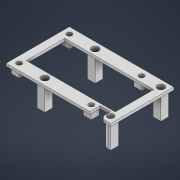
# Autodesk Inventor part: Adapter_Spannungswandler
Saved by Autodesk Inventor 2021 (Build 250183000, 183)
## iProperties
Created: 2021-02-07
Part Number: Adapter_Spannungswandler
Material: Generisch
Document SubType Name: Modeling
Designer: Ctroi
Density: 1 g/cm^3
Appearance: Vorgabe
Author: Ctroi
Autodesk Inventor part; units mm, degrees
ref_plane "YZ Plane" through (0, 0, 0) normal (1, 0, 0) x (0, 1, 0)
ref_plane "XZ Plane" through (0, 0, 0) normal (0, 1, 0) x (-1, 0, 0)
ref_plane "XY Plane" through (0, 0, 0) normal (0, 0, 1) x (1, 0, 0)
sketch "Skizze1" plane through (0, 0, 0) normal (0, 1, 0) x (-1, 0, 0)
  line L0 (28.5, 22.5) -> (-28.5, 22.5)
  line L1 (-28.5, 22.5) -> (-28.5, -22.5)
  line L2 (-28.5, -22.5) -> (28.5, -22.5)
  line L3 (28.5, -22.5) -> (28.5, 22.5)
  line L4 (-39.9, 0) -> (39.9, 0) projected
  line L5 (0, -31.5) -> (0, 31.5) projected
  circle A0 centre (-25.5, 19.5) radius 1.6
  circle A1 centre (25.5, 19.5) radius 1.6
  circle A2 centre (25.5, -19.5) radius 1.6
  circle A3 centre (-25.5, -19.5) radius 1.6
  line L6 (-28.5, 22.5) -> (-22.5, 22.5)
  line L7 (-22.5, 22.5) -> (-22.5, 16.5)
  line L8 (-22.5, 16.5) -> (-28.5, 16.5)
  line L9 (-28.5, 16.5) -> (-28.5, 22.5)
  line L10 (-14.5, 22.5) -> (-22.5, 22.5)
  line L11 (-22.5, 22.5) -> (-22.5, 16.5)
  line L12 (-22.5, 16.5) -> (-14.5, 16.5)
  line L13 (-14.5, 16.5) -> (-14.5, 22.5)
  line L14 (-28.5, -22.5) -> (-22.5, -22.5)
  line L15 (-22.5, -22.5) -> (-22.5, -16.5)
  line L16 (-22.5, -16.5) -> (-28.5, -16.5)
  line L17 (-28.5, -16.5) -> (-28.5, -22.5)
  line L18 (28.5, -22.5) -> (22.5, -22.5)
  line L19 (22.5, -22.5) -> (22.5, -16.5)
  line L20 (22.5, -16.5) -> (28.5, -16.5)
  line L21 (28.5, -16.5) -> (28.5, -22.5)
  line L22 (28.5, 22.5) -> (22.5, 22.5)
  line L23 (22.5, 22.5) -> (22.5, 16.5)
  line L24 (22.5, 16.5) -> (28.5, 16.5)
  line L25 (28.5, 16.5) -> (28.5, 22.5)
  point P0 (0, 0)
  dimension "d0" = 57
  dimension "d1" = 45
  dimension "d2" = 3.2
  dimension "d3" = 3.2
  dimension "d4" = 3.2
  dimension "d5" = 3.2
  dimension "d6" = 39
  dimension "d7" = 19.5
  dimension "d8" = 51
  dimension "d9" = 51
  dimension "d10" = 39
  dimension "d11" = 19.5
  dimension "d13" = 3
  dimension "d14" = 25.5
  dimension "d15" = 6
  dimension "d16" = 6
  dimension "d17" = 0
  dimension "d18" = 8
  dimension "d19" = 6
  dimension "d20" = 6
  dimension "d21" = 6
  dimension "d22" = 6
  dimension "d23" = 6
  dimension "d24" = 6
  constraints: 48 end point, 12 parallel, 6 horizontal, 6 perpendicular, 4 centre point, 2 point on line, 2 other
  measures "d0" distance of L2.end L1.end
  measures "d1" distance of L1.end L0.end
  measures "d2" diameter of A0
  measures "d3" diameter of A1
  measures "d4" diameter of A2
  measures "d5" diameter of A3
  measures "d6" distance of A2.centre A1.centre
  measures "d7" distance from line of L4 A1.centre
  measures "d8" distance of A0.centre A1.centre
  measures "d9" distance of A3.centre A2.centre
  measures "d10" distance of A3.centre A0.centre
  measures "d11" distance from line of L4 A0.centre
  measures "d13" distance from line of L2 A2.centre
  measures "d14" distance from line of L5 A1.centre
  measures "d15" distance of L7.end L8.end
  measures "d16" distance of L6.end L7.end
  measures "d17" distance between parallel lines of L7 L11
  measures "d18" distance between parallel lines of L7 L13
  measures "d19" distance of L16.end L15.end
  measures "d20" distance of L15.end L14.end
  measures "d21" distance of L19.end L20.end
  measures "d22" distance of L18.end L19.end
  measures "d23" distance of L24.end L23.end
  measures "d24" distance of L23.end L22.end
extrude "Extrusion1" add sketch "Skizze1" along normal blind 2 and the other way blind 23 contours L3 L24 L23 L0 | L3 L2 L19 L20 | L7 L8 L1 L0 | L16 L15 L2 L1
extrude "Extrusion2" add sketch "Skizze1" along normal blind 2 contours L23 L24 L3 L4 L5 L0 | L5 L4 L1 L8 L12 L13 L0 | L3 L20 L19 L2 L5 L4 | L5 L2 L15 L16 L1 L4
sketch "Skizze2" plane through (-28.5, -23, 22.5) normal (-1, 0, 0) x (0, 0, 1)
  line L0 (0, 0) -> (0, 25) projected
  line L1 (-45, 0) -> (-45, 25) projected
  line L2 (0, 25) -> (-45, 25)
  line L3 (-45, 25) -> (-45, 23)
  line L4 (-45, 23) -> (0, 23)
  line L5 (0, 23) -> (0, 25)
  point P0 (-22.5, 23)
  constraints: 8 end point, 2 parallel, 1 horizontal, 1 perpendicular, 1 point on line
extrude "Extrusion3" add sketch "Skizze2" along normal blind 20
sketch "Skizze4" plane through (0, 0, 0) normal (0, -1, 0) x (1, 0, 0)
  line L0 (-48.5, 22.5) -> (-48.5, -22.5) projected
  line L1 (-48.5, -22.5) -> (-42.5, -22.5)
  line L2 (-42.5, -22.5) -> (-42.5, -16.5)
  line L3 (-42.5, -16.5) -> (-48.5, -16.5)
  line L4 (-48.5, -16.5) -> (-48.5, -22.5)
  line L5 (-48.5, 22.5) -> (-42.5, 22.5)
  line L6 (-42.5, 22.5) -> (-42.5, 16.5)
  line L7 (-42.5, 16.5) -> (-48.5, 16.5)
  line L8 (-48.5, 16.5) -> (-48.5, 22.5)
  line L9 (22.5, -22.5) -> (-22.5, -22.5) projected
  line L10 (7.5, -22.5) -> (13.5, -22.5)
  line L11 (13.5, -22.5) -> (13.5, -16.5)
  line L12 (13.5, -16.5) -> (7.5, -16.5)
  line L13 (7.5, -16.5) -> (7.5, -22.5)
  line L14 (28.5, 16.5) -> (28.5, -16.5) projected
  line L15 (-22.5, 22.5) -> (14.5, 22.5) projected
  line L16 (13.5, 22.5) -> (7.5, 22.5)
  line L17 (7.5, 22.5) -> (7.5, 16.5)
  line L18 (7.5, 16.5) -> (13.5, 16.5)
  line L19 (13.5, 16.5) -> (13.5, 22.5)
  line L20 (28.5, 16.5) -> (28.5, 22.5) projected
  point P0 (0, 0)
  dimension "d45" = 6
  dimension "d46" = 6
  dimension "d47" = 6
  dimension "d48" = 6
  dimension "d49" = 6
  dimension "d50" = 6
  dimension "d51" = 15
  dimension "d52" = 6
  dimension "d53" = 6
  dimension "d54" = 15
  constraints: 32 end point, 8 parallel, 4 horizontal, 4 perpendicular, 2 point on line
  measures "d45" distance of L3.end L2.end
  measures "d46" distance of L2.end L1.end
  measures "d47" distance of L6.end L7.end
  measures "d48" distance of L5.end L6.end
  measures "d49" distance of L12.end L11.end
  measures "d50" distance of L11.end L10.end
  measures "d51" distance between parallel lines of L14 L11
  measures "d52" distance of L18.end L17.end
  measures "d53" distance of L17.end L16.end
  measures "d54" distance between parallel lines of L20 L19
extrude "Extrusion4" add sketch "Skizze4" along normal blind 5
sketch "Skizze3" plane through (0, 2, 0) normal (0, 1, 0) x (1, 0, 0)
  circle A0 centre (10.5, -19.5) radius 2
  circle A1 centre (10.5, 19.5) radius 2
  line L0 (43.9, 0) -> (-63.9, 0) projected
  line L1 (28.5, -22.5) -> (28.5, 22.5) projected
  circle A2 centre (-45.5, -19.5) radius 2
  circle A3 centre (-45.5, 19.5) radius 2
  line L2 (14.5, -22.5) -> (-48.5, -22.5) projected
  line L3 (28.5, 22.5) -> (-48.5, 22.5) projected
  point P0 (0, 0)
  dimension "d33" = 4
  dimension "d34" = 4
  dimension "d35" = 39
  dimension "d36" = 19.5
  dimension "d37" = 18
  dimension "d38" = 18
  dimension "d39" = 4
  dimension "d40" = 4
  dimension "d41" = 3
  dimension "d42" = 3
  dimension "d43" = 56
  dimension "d44" = 56
  constraints: 4 centre point
  measures "d33" diameter of A0
  measures "d34" diameter of A1
  measures "d35" distance of A1.centre A0.centre
  measures "d36" distance from line of L0 A0.centre
  measures "d37" distance from line of L1 A0.centre
  measures "d38" distance from line of L1 A1.centre
  measures "d39" diameter of A2
  measures "d40" diameter of A3
  measures "d41" distance from line of L2 A2.centre
  measures "d42" distance from line of L3 A3.centre
  measures "d43" distance of A0.centre A2.centre
  measures "d44" distance of A1.centre A3.centre
extrude "Extrusion5" cut sketch "Skizze3" against normal blind 6
sketch "Skizze5" plane through (0, -23, 0) normal (0, -1, 0) x (1, 0, 0)
  circle A0 centre (-25.5, 19.5) radius 1.6 projected
  circle A1 centre (-25.5, 19.5) radius 1.6
  line L0 (-28.5, 22.5) -> (-22.5, 22.5)
  line L1 (-22.5, 22.5) -> (-22.5, 16.5)
  line L2 (-22.5, 16.5) -> (-28.5, 16.5)
  line L3 (-28.5, 16.5) -> (-28.5, 22.5)
  line L4 (22.5, 16.5) -> (28.5, 16.5) projected
  line L5 (22.5, 22.5) -> (28.5, 22.5) projected
  line L6 (28.5, 16.5) -> (22.5, 16.5)
  line L7 (22.5, 16.5) -> (22.5, 22.5)
  line L8 (22.5, 22.5) -> (28.5, 22.5)
  line L9 (28.5, 22.5) -> (28.5, 16.5)
  circle A2 centre (25.5, 19.5) radius 1.6
  circle A3 centre (25.5, -19.5) radius 1.6 projected
  circle A4 centre (25.5, -19.5) radius 1.6
  line L10 (28.5, -22.5) -> (-48.5, -22.5) projected
  line L11 (22.5, -16.5) -> (22.5, -22.5) projected
  line L12 (28.5, -22.5) -> (22.5, -22.5)
  line L13 (22.5, -22.5) -> (22.5, -16.5)
  line L14 (22.5, -16.5) -> (28.5, -16.5)
  line L15 (28.5, -16.5) -> (28.5, -22.5)
  line L16 (-28.5, -16.5) -> (-28.5, -22.5) projected
  line L17 (-22.5, -22.5) -> (-28.5, -22.5)
  line L18 (-28.5, -22.5) -> (-28.5, -16.5)
  line L19 (-28.5, -16.5) -> (-22.5, -16.5)
  line L20 (-22.5, -16.5) -> (-22.5, -22.5)
  circle A5 centre (-25.5, -19.5) radius 1.6 projected
  circle A6 centre (-25.5, -19.5) radius 1.6
  point P0 (0, 0)
  dimension "d59" = 3.2
  dimension "d60" = 3.2
  dimension "d61" = 3.2
  dimension "d62" = 3.2
  dimension "d63" = 3
  dimension "d64" = 3
  constraints: 32 end point, 8 parallel, 4 centre point, 4 horizontal, 4 perpendicular, 3 coincident, 1 point on line
  measures "d59" diameter of A1
  measures "d60" diameter of A2
  measures "d61" diameter of A4
  measures "d62" diameter of A6
  measures "d63" distance from line of L5 A2.centre
  measures "d64" distance from line of L9 A2.centre
extrude "Extrusion6" cut sketch "Skizze5" against normal blind 5
sketch "Skizze6" plane through (0, 2, 0) normal (0, 1, 0) x (1, 0, 0)
  line L0 (-44.5, 15) -> (24.5, 15)
  line L1 (24.5, 15) -> (24.5, -15)
  line L2 (24.5, -15) -> (-44.5, -15)
  line L3 (-44.5, -15) -> (-44.5, 15)
  line L4 (43.9, 0) -> (-63.9, 0) projected
  line L5 (28.5, -22.5) -> (28.5, 22.5) projected
  point P0 (0, 0)
  dimension "d67" = 69
  dimension "d68" = 30
  dimension "d69" = 4
  constraints: 8 end point, 2 parallel, 1 horizontal, 1 perpendicular, 1 other
  measures "d67" distance of L1.end L2.end
  measures "d68" distance of L0.end L1.end
  measures "d69" distance between parallel lines of L5 L1
extrude "Extrusion7" cut sketch "Skizze6" against normal up to surface (2 mm away)
sketch "Skizze8" plane through (14.5, 0, 22.5) normal (0, 0, 1) x (1, 0, 0)
  line L0 (-63, 2) -> (-63, -5) projected
  line L1 (10, 0) -> (-59, 0) projected
  line L2 (-63, 2) -> (0, 2)
  line L3 (0, 2) -> (0, 0)
  line L4 (0, 0) -> (-63, 0)
  line L5 (-63, 0) -> (-63, 2)
  line L6 (8, 0) -> (14, 0) projected
  line L7 (14, 0) -> (8, 0)
  line L8 (8, 0) -> (8, 2)
  line L9 (8, 2) -> (14, 2)
  line L10 (14, 2) -> (14, 0)
  line L11 (8, 2) -> (14, 2) projected
  point P0 (-14.5, 0)
  point P1 (-63, 0)
  point P2 (-59, 0)
  point P3 (8, 0)
  dimension "d73" = 63
  dimension "d74" = 6
  dimension "d75" = 0
  constraints: 16 end point, 4 parallel, 2 horizontal, 2 perpendicular, 1 point on line
  measures "d73" distance of L3.end L4.end
  measures "d74" distance of L8.end L9.end
  measures "d75" distance between parallel lines of L11 L9
extrude "Extrusion8" add sketch "Skizze8" along normal blind 2
sketch "Skizze9" plane through (28.5, 2, -22.5) normal (0, 0, -1) x (-1, 0, 0)
  line L0 (0, 0) -> (6, 0) projected
  line L1 (77, -2) -> (77, -7) projected
  line L2 (0, 0) -> (77, 0)
  line L3 (77, 0) -> (77, -2)
  line L4 (77, -2) -> (0, -2)
  line L5 (0, -2) -> (0, 0)
  point P0 (28.5, -2)
  constraints: 8 end point, 2 parallel, 1 horizontal, 1 perpendicular
extrude "Extrusion9" add sketch "Skizze9" along normal blind 2
sketch "Skizze7" plane through (0, 2, 0) normal (0, 1, 0) x (1, 0, 0)
  circle A0 centre (-25.5, -19.5) radius 1.6 projected
  circle A1 centre (-25.5, -19.5) radius 2.75
  circle A2 centre (25.5, -19.5) radius 1.6 projected
  circle A3 centre (25.5, -19.5) radius 2.5
  circle A4 centre (25.5, 19.5) radius 1.6 projected
  circle A5 centre (25.5, 19.5) radius 2.75
  circle A6 centre (-25.5, 19.5) radius 1.6 projected
  circle A7 centre (-25.5, 19.5) radius 2.75
  point P0 (0, 0)
  dimension "d72" = 5.5
  dimension "d80" = 5
  dimension "d81" = 5.5
  dimension "d82" = 5.5
  constraints: 4 centre point, 4 coincident
  measures "d72" diameter of A1
  measures "d80" diameter of A3
  measures "d81" diameter of A5
  measures "d82" diameter of A7
sketch "Skizze10" plane through (28.5, 0, 16.5) normal (1, 0, 0) x (0, 0, -1)
  line L0 (41, 2) -> (-8, 2) projected
  line L1 (39, 0) -> (41, 0) projected
  line L2 (-8, 2) -> (41, 2)
  line L3 (41, 2) -> (41, 0)
  line L4 (41, 0) -> (-8, 0)
  line L5 (-8, 0) -> (-8, 2)
  point P0 (16.5, 0)
  constraints: 8 end point, 2 parallel, 1 horizontal, 1 perpendicular
extrude "Extrusion10" add sketch "Skizze10" along normal blind 2
sketch "Skizze11" plane through (-48.5, -23, 22.5) normal (-1, 0, 0) x (0, 0, 1)
  line L0 (-47, 25) -> (2, 25) projected
  line L1 (2.0117, 23) -> (-47, 23)
  line L2 (-47, 23) -> (-47, 25)
  line L3 (-47, 25) -> (2.0117, 25)
  line L4 (2.0117, 25) -> (2.0117, 23)
  point P0 (-22.5, 23)
  point P1 (2, 25)
  constraints: 8 end point, 2 parallel, 1 horizontal, 1 perpendicular
extrude "Extrusion11" add sketch "Skizze11" along normal blind 2
extrude "Extrusion12" cut sketch "Skizze7" against normal blind 4
fillet "Rundung1" radius 4 2 edges at (22.5, -9, 22.5) (22.5, 1, 24.5)
